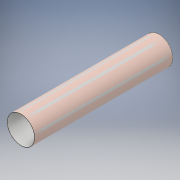
# Autodesk Inventor part: 零件1
Saved by Autodesk Inventor 2018.2 (Build 222227000, 227)
## iProperties
Created: 2018-07-04
Part Number: 零件1
Material: 常规
Document SubType Name: Modeling
Designer: Administrator
Density: 1 g/cm^3
Appearance: 默认
Author: Administrator
Autodesk Inventor part; units mm, degrees
ref_plane "YZ Plane" through (0, 0, 0) normal (1, 0, 0) x (0, 1, 0)
ref_plane "XZ Plane" through (0, 0, 0) normal (0, 1, 0) x (-1, 0, 0)
ref_plane "XY Plane" through (0, 0, 0) normal (0, 0, 1) x (1, 0, 0)
sketch "草图1" plane through (0, 0, 0) normal (0, 1, 0) x (-1, 0, 0)
  circle A0 centre (0, 0) radius 600
  dimension "d0" = 1200
  constraints: 1 centre point, 1 coincident
  measures "d0" diameter of A0
surface extrude "拉伸曲面1" sketch "草图1" along normal blind 6000 shown yes curves A0
thicken "加厚1" operation new thickness 12 both sides no extend neighbours no toward (0.9998154, 0, 0.0192135) faces at (-599.8892, 4000, -11.5281)
body "Srf1"
